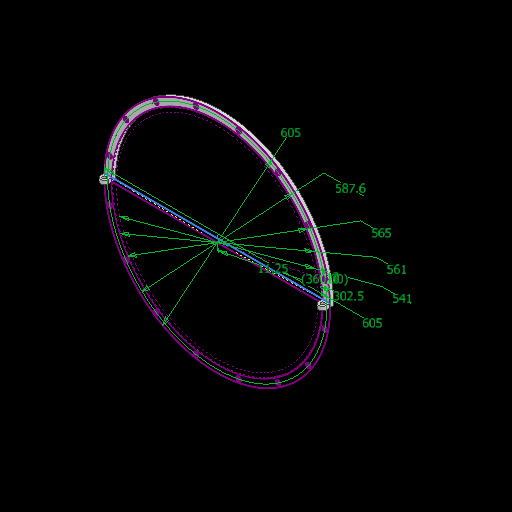
# Autodesk Inventor part: half_ring_1
Saved by Autodesk Inventor 2026.1 (Build 301233000, 233)
## iProperties
Created: 2025-09-17
Part Number: half_ring_1
Material: Generic
Document SubType Name: Modeling
Designer: drago
Density: 1 g/cm^3
Appearance: Default
Author: drago
Autodesk Inventor part; units mm, degrees
ref_plane "YZ Plane" through (0, 0, 0) normal (1, 0, 0) x (0, 1, 0)
ref_plane "XZ Plane" through (0, 0, 0) normal (0, 1, 0) x (-1, 0, 0)
ref_plane "XY Plane" through (0, 0, 0) normal (0, 0, 1) x (1, 0, 0)
sketch "Sketch1" plane through (0, 0, 0) normal (0, 0, 1) x (1, 0, 0)
  circle A0 centre (0, 0) radius 302.5
  circle A1 centre (0, 0) radius 270.5 construction
  circle A2 centre (0, 0) radius 280.5 construction
  circle A3 centre (0, 0) radius 282.5
  line L0 (-302.5, 0) -> (302.5, 0)
  circle A4 centre (0, 0) radius 293.8 construction
  line L1 (0, 0) -> (302.3347, 10) construction
  line L2 (0, 0) -> (-302.3347, 10) construction
  line L3 (0, 0) -> (293.8, 0) construction
  line L4 (0, 0) -> (296.6875, 59.0148) construction
  line L5 (0, 0) -> (302.5, 0) construction
  circle A5 centre (288.1547, 57.3175) radius 5 construction
  circle A6 centre (288.1547, 57.3175) radius 6
  circle A7 centre (244.2858, 163.2265) radius 6
  circle A8 centre (244.2858, 163.2265) radius 5 construction
  circle A9 centre (163.2265, 244.2858) radius 6
  circle A10 centre (163.2265, 244.2858) radius 5 construction
  circle A11 centre (57.3175, 288.1547) radius 6
  circle A12 centre (57.3175, 288.1547) radius 5 construction
  circle A13 centre (-57.3175, 288.1547) radius 6
  circle A14 centre (-57.3175, 288.1547) radius 5 construction
  circle A15 centre (-163.2265, 244.2858) radius 6
  circle A16 centre (-163.2265, 244.2858) radius 5 construction
  circle A17 centre (-244.2858, 163.2265) radius 6
  circle A18 centre (-244.2858, 163.2265) radius 5 construction
  circle A19 centre (-288.1547, 57.3175) radius 6
  circle A20 centre (-288.1547, 57.3175) radius 5 construction
  circle A21 centre (-288.1547, -57.3175) radius 6
  circle A22 centre (-288.1547, -57.3175) radius 5 construction
  circle A23 centre (-244.2858, -163.2265) radius 6
  circle A24 centre (-244.2858, -163.2265) radius 5 construction
  circle A25 centre (-163.2265, -244.2858) radius 6
  circle A26 centre (-163.2265, -244.2858) radius 5 construction
  circle A27 centre (-57.3175, -288.1547) radius 6
  circle A28 centre (-57.3175, -288.1547) radius 5 construction
  circle A29 centre (57.3175, -288.1547) radius 6
  circle A30 centre (57.3175, -288.1547) radius 5 construction
  circle A31 centre (163.2265, -244.2858) radius 6
  circle A32 centre (163.2265, -244.2858) radius 5 construction
  circle A33 centre (244.2858, -163.2265) radius 6
  circle A34 centre (244.2858, -163.2265) radius 5 construction
  circle A35 centre (288.1547, -57.3175) radius 6
  circle A36 centre (288.1547, -57.3175) radius 5 construction
  line L6 (-302.3347, 10) -> (302.3347, 10)
  point P0 (282.5, 0)
  point P1 (302.5, 0)
  point P2 (-282.5, 0)
  point P3 (-282.3456, 9.3388)
  point P4 (282.3456, 9.3388)
  point P5 (282.323, 10)
  point P6 (-282.323, 10)
  dimension "d5" = 587.6
  dimension "d0" = 605
  dimension "d1" = 541
  dimension "d2" = 561
  dimension "d3" = 565
  dimension "d4" = 605
  dimension "d36" = 302.5
  dimension "d37" = 11.25
  dimension "d38" = 10
  dimension "d39" = 12
  dimension "d42" = 360
  constraints: 36 centre point, 22 coincident, 14 end point, 4 horizontal, 2 point on circle, 1 equal length, 1 midpoint, 1 point on line, 68 other
  measures "d0" diameter of A0
  measures "d1" diameter of A1
  measures "d2" diameter of A2
  measures "d3" diameter of A3
  measures "d4" distance of L0.start L0.end
  measures "d36" distance of L3.start L4.end
  measures "d37" angle of L5 L4
  measures "d38" diameter of A5
  measures "d39" diameter of A6
extrude "Extrusion4" add sketch "Sketch1" against normal blind 10 contours L0 A3 L6 A0 | L6 A3 A0 | A0 L6 A3 L0
extrude "Extrusion5" add sketch "Sketch1" along normal blind 20 contours L0 A3 L6 A0 | A0 L6 A3 L0
sketch "Sketch3" plane through (-302.5, 0, -10) normal (0, -1, 0) x (1, 0, 0)
  circle A0 centre (10, 20) radius 5
  line L0 (0, 30) -> (20, 30) projected
  line L1 (0, 30) -> (0, 0) projected
  line L2 (20, 0) -> (20, 30) projected
  circle A1 centre (595, 20) radius 5
  line L3 (585, 30) -> (605, 30) projected
  line L4 (605, 0) -> (605, 30) projected
  line L5 (585, 0) -> (585, 30) projected
  point P0 (302.5, 10)
  dimension "d50" = 10
  dimension "d51" = 10
  dimension "d52" = 10
  dimension "d53" = 10
  dimension "d54" = 10
  dimension "d55" = 10
  constraints: 2 centre point
  measures "d50" diameter of A0
  measures "d51" distance from line of L0 A0.centre
  measures "d52" distance from line of L1 A0.centre
  measures "d53" diameter of A1
  measures "d54" distance from line of L3 A1.centre
  measures "d55" distance from line of L4 A1.centre
full round fillet "Full Round Fillet2" first side at (302.4816, 3.3339, 3.3333) centre faces at (-289.0263, 8.8891, 20) second side at (282.4803, 3.334, 3.3333)
full round fillet "Full Round Fillet3" first side at (302.4816, 3.3339, 3.3333) centre faces at (289.0263, 8.8891, 20) second side at (282.4803, 3.334, 3.3333)
hole "Hole2" at (-292.5, 0, 10) at (292.5, 0, 10) direction (0, 1, 0) diameter 10 end through all
body "Solid2"
